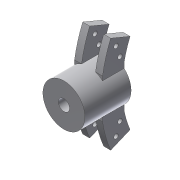
# Autodesk Inventor part: M02 - Main Spherical Shaft
Saved by Autodesk Inventor 2016 (Build 200138000, 138)
## iProperties
Created: 2016-12-26
Part Number: M02 - Main Spherical Shaft
Material: ABS Plastic
Document SubType Name: Modeling
Designer: Fernando
Stock Number: 0
Mass: 28.9592 g
Surface Area: 86.5698 cm^2
Volume: 27.32 cm^3
Density: 1.06 g/cm^3
Appearance: Smooth - White
SurfaceArea_m2: .01
Author: Fernando
Autodesk Inventor part; units mm, degrees
ref_plane "YZ Plane" through (0, 0, 0) normal (1, 0, 0) x (0, 1, 0)
ref_plane "XY Plane" through (0, 0, 0) normal (0, 0, 1) x (1, 0, 0)
sketch "Sketch2" plane through (0, 0, 0) normal (0, 1, 0) x (-1, 0, 0)
  circle A0 centre (0, 0) radius 15
  circle A1 centre (0, 0) radius 4
  dimension "d11" = 8
  dimension "d12" = 30
  constraints: 2 centre point, 2 coincident
  measures "d11" diameter of A1
  measures "d12" diameter of A0
extrude "Extrusion2" add sketch "Sketch2" along normal blind 33
sketch "Sketch3" plane through (0, 33, 0) normal (0, 1, 0) x (1, 0, 0)
  line L0 (-3.4641, 2) -> (3.4641, 2)
  arc A0 (3.4641, 2) -> (-3.4641, 2) centre (0, 0) ccw
  circle A1 centre (0, 0) radius 4 projected
  dimension "d15" = 2
  constraints: 2 end point, 2 point on circle, 1 centre point, 1 coincident, 1 concentric, 1 horizontal
  measures "d15" distance from line of L0 point (0, 0)
extrude "Extrusion3" add sketch "Sketch3" against normal blind 6 contours A0 L0
sketch "Sketch4" plane through (0, 0, 0) normal (1, 0, 0) x (0, 1, 0)
  line L0 (33, -15) -> (33, 15) projected
  arc A0 (33, -15) -> (179.9694, -15) centre (106.4847, 0) ccw
  arc A1 (179.9694, 15) -> (33, 15) centre (106.4847, 0) ccw
  line L1 (179.9694, -15) -> (179.9694, 15)
  line L2 (179.9694, 0) -> (0, 0) construction
  arc A2 (194.9694, 16.4456) -> (17.4285, 13) centre (106.4847, 0) ccw
  arc A3 (17.4285, -13) -> (194.9694, -16.4456) centre (106.4847, 0) ccw
  line L3 (194.9694, -16.4456) -> (194.9694, 16.4456)
  line L4 (33, -15) -> (33, -13)
  line L5 (17.4285, -13) -> (33, -13)
  line L6 (33, 15) -> (33, 13)
  line L7 (33, 13) -> (17.4285, 13)
  dimension "d18" = 30
  dimension "d19" = 75
  dimension "d21" = 15
  dimension "d22" = 15
  dimension "d25" = 2
  constraints: 14 end point, 11 point on circle, 4 centre point, 4 concentric, 3 horizontal, 2 point on line, 2 vertical, 1 midpoint, 1 parallel, 1 perpendicular
  measures "d18" distance of L1.start L1.end
  measures "d19" radius of A1
  measures "d21" radial gap between concentric circles of A0 A3
  measures "d22" distance between parallel lines of L1 L3
  measures "d25" distance from line of L0.start L5
extrude "Extrusion4" add sketch "Sketch4" along normal mid plane 10 contours A0 L1 A1 L0 L7 A2 L3 A3 L5
sketch "Sketch5" plane through (0, 0, 0) normal (1, 0, 0) x (0, 1, 0)
  line L0 (192.944, -40.3167) -> (106.4847, 0) construction
  arc A0 (33, -15) -> (179.9694, -15) centre (106.4847, 0) ccw projected
  line L1 (106.4847, 0) -> (8.9056, -48.1461) construction
  line L2 (106.4847, 0) -> (191.7041, -48.7426) construction
  line L3 (106.4847, 0) -> (209.5292, 0) construction
  line L4 (188.143, -38.0779) -> (187.0653, -40.389)
  line L5 (187.0653, -40.389) -> (182.5338, -38.2759)
  line L6 (182.5338, -38.2759) -> (182.3859, -38.5931)
  line L7 (182.3859, -38.5931) -> (168.7913, -32.2538)
  line L8 (168.7913, -32.2538) -> (170.0169, -29.6255)
  line L9 (188.143, -38.0779) -> (170.0169, -29.6255)
  point P0 (0, 0)
  dimension "d26" = 128.738
  dimension "d27" = 4.768
  dimension "d28" = 25
  dimension "d29" = 90.1
  dimension "d30" = 5
  dimension "d31" = 15
  dimension "d32" = 5.1
  dimension "d33" = 5.8
  constraints: 20 end point, 4 perpendicular, 2 point on line, 1 coincident, 1 horizontal
  measures "d26" angle of L1 L0
  measures "d27" angle of L0 L2
  measures "d28" angle of L3 L0
  measures "d29" distance of L0.end L4.start
  measures "d30" distance of L4.end L5.end
  measures "d31" distance of L6.end L7.end
  measures "d32" diameter of L5 L0
  measures "d33" diameter of L7 L0
revolve "Revolution1" cut sketch "Sketch5" angle 360 about axis through (0, 192.944, -40.3167) along (0, -0.9063078, 0.4226183)
pattern_circular "Circular Pattern1" count 26 over 128.73 about axis through (0, 106.4847, 0) along (-1, 0, 0) of "Revolution1"
sketch "Sketch6" plane through (-5, 179.9694, -15) normal (0, -1, 0) x (1, 0, 0)
  circle A0 centre (5, 15) radius 15
  dimension "d38" = 30
  constraints: 1 centre point, 1 coincident
  measures "d38" diameter of A0
extrude "Extrusion5" add sketch "Sketch6" against normal blind 25
sketch "Sketch7" plane through (0, 204.9694, 0) normal (0, 1, 0) x (1, 0, 0)
  circle A0 centre (0, 0) radius 6
  dimension "d41" = 12
  constraints: 1 centre point, 1 coincident
  measures "d41" diameter of A0
extrude "Extrusion6" add sketch "Sketch7" along normal blind 25
sketch "Sketch8" plane through (0, 0, 0) normal (1, 0, 0) x (0, 1, 0)
  line L0 (71.4847, 25) -> (141.4847, 25)
  line L1 (141.4847, 25) -> (141.4847, -25)
  line L2 (141.4847, -25) -> (71.4847, -25)
  line L3 (71.4847, -25) -> (71.4847, 25)
  line L4 (71.4847, 25) -> (141.4847, -25) construction
  line L5 (141.4847, 25) -> (71.4847, -25) construction
  arc A0 (33, -15) -> (179.9694, -15) centre (106.4847, 0) ccw projected
  point P0 (0, 0)
  dimension "d44" = 70
  dimension "d45" = 50
  constraints: 12 end point, 2 midpoint, 2 parallel, 1 coincident, 1 horizontal, 1 horizontal alignment, 1 perpendicular
  measures "d44" distance of L1.end L2.end
  measures "d45" distance of L0.end L1.end
extrude "Extrusion7" add sketch "Sketch8" against normal up to surface (5 mm away)
sketch "Sketch10" plane through (0, 0, 0) normal (1, 0, 0) x (0, 1, 0)
  line L0 (179.9694, -14.1421) -> (179.9694, 14.1421) construction
  arc A0 (178.3965, 21.3002) -> (178.3965, -21.3002) centre (191.4847, 0) ccw
  arc A1 (33, -15) -> (179.9694, -15) centre (106.4847, 0) ccw construction
  arc A2 (179.9694, 15) -> (33, 15) centre (106.4847, 0) ccw construction
  arc A3 (178.3965, -21.3002) -> (178.3965, 21.3002) centre (106.4847, 0) ccw
  line L1 (71.4847, -25) -> (71.4847, 25) construction
  line L2 (141.4847, 25) -> (141.4847, -25) construction
  line L3 (37.2754, -28.8977) -> (71.4847, -25)
  line L4 (71.4847, -25) -> (71.4847, -15)
  line L5 (71.4847, -15) -> (33, -15)
  line L6 (71.4847, 25) -> (71.4847, 15)
  line L7 (33, 15) -> (71.4847, 15)
  line L8 (71.4847, 25) -> (37.2754, 28.8977)
  arc A4 (37.2754, 28.8977) -> (33, 15) centre (106.4847, 0) ccw
  arc A5 (33, -15) -> (37.2754, -28.8977) centre (106.4847, 0) ccw
  line L9 (141.4847, 25) -> (167.4355, 6.8291)
  line L10 (141.4847, -25) -> (167.4355, -6.8291)
  line L11 (141.4847, 25) -> (141.4847, -25)
  point P0 (0, 0)
  dimension "d51" = 25
  dimension "d52" = 85
  dimension "d53" = 6.5
  dimension "d54" = 6.5
  dimension "d55" = 55
  dimension "d56" = 55
  constraints: 18 end point, 14 point on circle, 4 centre point, 2 concentric, 2 point on line, 1 horizontal, 1 horizontal alignment, 1 perpendicular, 1 vertical
  measures "d51" radius of A0
  measures "d52" distance of A1.centre A0.centre
  measures "d53" angle of L5 L3
  measures "d54" angle of L8 L7
  measures "d55" angle of L2 L9
  measures "d56" angle of L2 L10
extrude "Extrusion8" add sketch "Sketch10" along normal mid plane 10
fillet "Fillet1" radius 5 2 edges at (0, 167.4355, 6.8291) (0, 167.4355, -6.8291)
chamfer "Chamfer1" distance 2 angle 45 1 edges at (-6, 229.9694, 0)
sketch "Sketch11" plane through (5, 0, 0) normal (1, 0, 0) x (0, 0, -1)
  arc A0 (28.8977, 37.2754) -> (21.3002, 178.3965) centre (0, 106.4847) ccw projected
  arc A1 (14.1421, 17.6027) -> (16.4456, 194.9694) centre (0, 106.4847) ccw projected
  point P0 (0, 0)
  point P1 (20, 30.0583)
  point P2 (28, 27.2887)
  dimension "d64" = 20
  dimension "d65" = 28
  dimension "d67" = 79
  dimension "d68" = 84
  measures "d64" horizontal distance of point (0, 0) point (20, 30.058)
  measures "d65" horizontal distance of point (0, 0) point (28, 27.289)
  measures "d67" distance of A0.centre point (20, 30.058)
  measures "d68" distance of A0.centre point (28, 27.289)
hole "Hole1" at (5, 30.0583, -20) at (5, 27.2887, -28) direction (-1, 0, 0) diameter 3.2 end through all
ref_plane "Work Plane1" through (0, 106.4847, 0) normal (0, 1, 0) x (1, 0, 0)
mirror "Mirror1" about plane through (0, 106.4847, 0) normal (0, 1, 0) of "Hole1"
mirror "Mirror2" about plane through (0, 0, 0) normal (0, 0, 1) of "Hole1", "Mirror1"
sketch "Sketch12" plane through (0, 0, 0) normal (1, 0, 0) x (0, 1, 0)
  arc A0 (178.3965, 21.3002) -> (37.2754, 28.8977) centre (106.4847, 0) ccw projected
  arc A1 (37.2754, -28.8977) -> (178.3965, -21.3002) centre (106.4847, 0) ccw projected
  arc A2 (194.9694, 16.4456) -> (17.6027, 14.1421) centre (106.4847, 0) ccw projected
  line L0 (37.2754, 28.8977) -> (23.4335, 34.6772)
  arc A3 (17.6027, -14.1421) -> (194.9694, -16.4456) centre (106.4847, 0) ccw projected
  line L1 (37.2754, -28.8977) -> (23.4335, -34.6772)
  line L2 (33, -14.1421) -> (33, 14.1421) projected
  arc A4 (37.2754, 28.8977) -> (33, 15) centre (106.4847, 0) ccw
  arc A5 (33, -15) -> (37.2754, -28.8977) centre (106.4847, 0) ccw
  line L3 (0, 15) -> (17.7435, 15) projected
  line L4 (0, -15) -> (17.7435, -15) projected
  line L5 (0, -15) -> (0, 15)
  line L6 (0, 15) -> (17.7435, 15)
  line L7 (0, -15) -> (17.7435, -15)
  line L8 (33, 15) -> (33, -15)
  arc A6 (23.4335, 34.6772) -> (17.7435, 15) centre (106.4847, 0) ccw
  arc A7 (17.7435, -15) -> (23.4335, -34.6772) centre (106.4847, 0) ccw
  point P0 (0, 0)
  constraints: 12 end point, 10 point on circle, 4 centre point, 4 concentric, 2 point on line, 1 collinear, 1 parallel, 1 perpendicular, 1 vertical
extrude "Extrusion9" cut sketch "Sketch12" along normal mid plane 50 keep common part
sketch "Sketch13" plane through (5, 0, 0) normal (1, 0, 0) x (0, 0, -1)
  arc A0 (-28.8977, 37.2754) -> (-15, 33) centre (0, 106.4847) ccw projected
  line L0 (-34.6772, 23.4335) -> (-28.8977, 37.2754) projected
  arc A1 (-34.6772, 23.4335) -> (-14.1421, 17.6027) centre (0, 106.4847) ccw projected
  line L1 (-14.1421, 33) -> (-14.1421, 17.6027) projected
  line L2 (-14.1421, 33) -> (-15, 33) projected
  circle A2 centre (-20, 30.0583) radius 1.6 projected
  circle A3 centre (-28, 27.2887) radius 1.6 projected
  arc A4 (15, 33) -> (28.8977, 37.2754) centre (0, 106.4847) ccw projected
  line L3 (15, 33) -> (14.1421, 33) projected
  line L4 (14.1421, 17.6027) -> (14.1421, 33) projected
  arc A5 (14.1421, 17.6027) -> (34.6772, 23.4335) centre (0, 106.4847) ccw projected
  line L5 (28.8977, 37.2754) -> (34.6772, 23.4335) projected
  circle A6 centre (20, 30.0583) radius 1.6 projected
  circle A7 centre (28, 27.2887) radius 1.6 projected
  line L6 (-14.1421, 33) -> (14.1421, 33)
  line L7 (14.1421, 17.6027) -> (-14.1421, 17.6027)
  point P0 (0, 0)
  constraints: 4 end point, 1 horizontal, 1 parallel
extrude "Extrusion10" add sketch "Sketch13" along normal blind 5
mirror "Mirror3" about plane through (0, 0, 0) normal (1, 0, 0) of "Extrusion10"
sketch "Sketch14" plane through (0, 33, 0) normal (0, 1, 0) x (1, 0, 0)
  circle A0 centre (0, 0) radius 15 construction
  arc A1 (-10, 11.1803) -> (-10, -11.1803) centre (0, 0) ccw construction
  line L0 (-5, -14.1421) -> (5, -14.1421) construction
  line L1 (5, -14.1421) -> (5, -46.8018)
  line L2 (5, -46.8018) -> (-5, -46.8018)
  line L3 (-5, -46.8018) -> (-5, -14.1421)
  line L4 (5, 14.1421) -> (-5, 14.1421) construction
  line L5 (-5, 14.1421) -> (-5, 41.5795)
  line L6 (-5, 41.5795) -> (5, 41.5795)
  line L7 (5, 41.5795) -> (5, 14.1421)
  line L8 (0, 14.1421) -> (0, -14.1421) construction
  arc A2 (-5, -14.1421) -> (5, -14.1421) centre (0, 0) ccw
  arc A3 (5, 14.1421) -> (-5, 14.1421) centre (0, 0) ccw
  dimension "d81" = 10
  constraints: 18 end point, 7 point on circle, 4 concentric, 4 parallel, 3 centre point, 2 horizontal, 2 midpoint, 2 perpendicular, 2 point on line, 1 coincident
  measures "d81" distance of L1.end L2.end
extrude "Extrusion11" cut sketch "Sketch14" along normal mid plane 50
ref_plane "Work Plane2" through (0, 0, 0) normal (1, 0, 0) x (0, 1, 0)
equation "\"d27\" = 0.037037 * d26"
body "Solid2"
